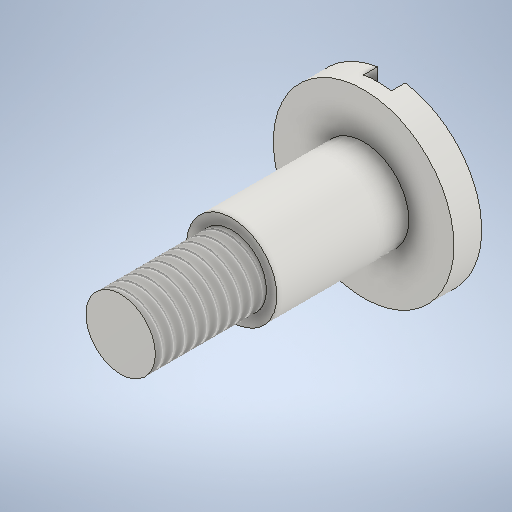
# Autodesk Inventor part: Crankpin
Saved by Autodesk Inventor 2025.2 (Build 292293000, 293)
## iProperties
Created: 2025-06-12
Part Number: Crankpin
Material: Steel AISI 1020 107 HR
Document SubType Name: Modeling
Designer: bless
Density: 7.87 g/cm^3
Appearance: Steel
Author: bless
Autodesk Inventor part; units mm, degrees
ref_plane "YZ Plane" through (0, 0, 0) normal (1, 0, 0) x (0, 1, 0)
ref_plane "XY Plane" through (0, 0, 0) normal (0, 0, 1) x (1, 0, 0)
sketch "Sketch1" plane through (0, 0, 0) normal (0, 0, 1) x (1, 0, 0)
  circle A0 centre (0, 0) radius 6.5
  dimension "d0" = 13
  constraints: 1 centre point, 1 coincident
  measures "d0" diameter of A0
extrude "Extrusion1" add sketch "Sketch1" along normal blind 2
sketch "Sketch2" plane through (0, 0, 2) normal (0, 0, 1) x (1, 0, 0)
  circle A0 centre (0, 0) radius 6.5 projected
  circle A1 centre (0, 0) radius 3.25
  dimension "d3" = 6.5
  constraints: 1 centre point, 1 coincident
  measures "d3" diameter of A1
extrude "Extrusion2" add sketch "Sketch2" along normal blind 9.5 contours A1
ref_plane "Work Plane1" through (0, 6.5, 0) normal (0, 1, 0) x (-1, 0, 0)
sketch "Sketch3" plane through (0, 6.5, 0) normal (0, 1, 0) x (-1, 0, 0)
  line L0 (6.5, 0) -> (-6.5, 0) projected
  line L1 (-1, 0) -> (1, 0)
  line L2 (1, 0) -> (1, 1)
  line L3 (1, 1) -> (-1, 1)
  line L4 (-1, 1) -> (-1, 0)
  point P0 (0, 0)
  point P1 (1, 0.5)
  point P2 (0, 0)
  dimension "d7" = 2
  dimension "d8" = 1
  dimension "d9" = 1
  constraints: 8 end point, 2 midpoint, 2 parallel, 1 horizontal, 1 perpendicular, 1 point on line
  measures "d7" distance from line of point (1, 0.5) L4
  measures "d8" distance between parallel lines of L3 L0
  measures "d9" distance from line of L2 point (0, 0)
extrude "Extrusion3" cut sketch "Sketch3" against normal through all
sketch "Sketch4" plane through (0, 0, 11.5) normal (0, 0, 1) x (1, 0, 0)
  circle A0 centre (0, 0) radius 3.25 projected
  circle A1 centre (0, 0) radius 2.5
  dimension "d12" = 5
  constraints: 1 centre point, 1 coincident
  measures "d12" diameter of A1
extrude "Extrusion4" add sketch "Sketch4" along normal blind 8 contours A1
thread "Thread1" size "M5x0.8" class "6g" standard "ANSI Metric M Profile" length 8
body "Solid1"
